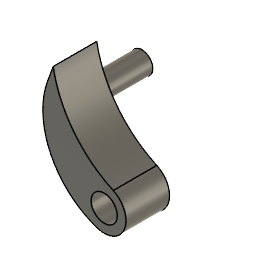
Pawl (Autodesk Fusion 360 design; units mm, degrees)
part number: 2026-05-26-15-53-21-879
Autodesk Fusion 360 part; units mm, degrees
sketch "ratchet scketch & pawl" plane through (0, 0, 0) normal (0, 1, 0) x (1, 0, 0)
  circle A0 centre (0, 0) radius 7.75 construction
  circle A1 centre (0, 0) radius 6.5 construction
  line L0 (0, 0) -> (1.3458, 7.6323) construction
  line L1 (0, 0) -> (-2.8494, 5.8422) construction
  arc A2 (1.3458, 7.6323) -> (-2.8494, 5.8422) centre (0.5379, 3.7147) ccw construction
  line L2 (0, 0) -> (6.5, 0) construction
  line L3 (0, 0) -> (4.4082, 25) construction
  circle A3 centre (2.9976, 17) radius 1.5
  circle A4 centre (2.9976, 17) radius 2.5
  line L4 (-2.8494, 5.8422) -> (-0.2045, 20.8422) construction
  line L5 (-2.8494, 5.8422) -> (-3.5335, 7.7215)
  arc A5 (4.0328, 14.7244) -> (-2.8494, 5.8422) centre (9.0259, 3.7482) ccw
  arc A6 (2.2215, 19.3765) -> (-3.5335, 7.7215) centre (5.0435, 10.7347) ccw
  circle A7 centre (-2.6702, 10.3422) radius 1.25
  dimension "d28" = 13
  dimension "d29" = 15.5
  dimension "d30" = 80
  dimension "d31" = 36
  dimension "d32" = 4
  dimension "d33" = 25
  dimension "d34" = 3
  dimension "d35" = 5
  dimension "d36" = 15
  dimension "d37" = 2
  dimension "d40" = 30
  dimension "d43" = 9.0909
  dimension "d44" = 17
  dimension "d45" = 2.5
  dimension "d46" = 4.5
  dimension "d47" = 7.7237
  constraint coincident A0.centre A1.centre
  constraint coincident A0 L0.end
  constraint coincident A1 L1.end
  constraint coincident A1 L2.end
  constraint horizontal L2
  constraint parallel L0 L3
  constraint coincident L3 A3.centre
  constraint concentric A3 A4
  constraint parallel L3 L4
  constraint tangent L4 A5
  constraint coincident A4 A5.start
  constraint coincident A4 A6.start
  constraint tangent A4 A5
  constraint tangent A4 A6
  measures "d28" diameter of A1
  measures "d29" diameter of A0
  measures "d30" angle of L0 L2
  measures "d31" angle of L0 L1
  measures "d32" radius of A2
  measures "d33" vertical distance of A0.centre L3.end
  measures "d34" diameter of A3
  measures "d35" diameter of A4
  measures "d36" vertical distance of L1.end L4.end
  measures "d37" distance of L1.end L5.end
  measures "d40" angle of L4 L5
  measures "d43" radius of A6
  measures "d44" vertical distance of A0.centre A3.centre
  measures "d45" diameter of A7
  measures "d46" vertical distance of L1.end A7.centre
  measures "d47" distance of A6.centre A7.centre
extrude "Extrude1" add sketch "ratchet scketch & pawl" along normal blind 5 contours A4 | A4 L5 A5 A6 | A7 makes body 1
move_body "Move1" bodies 1 to x (0, 0, 1) y (0, 1, 0) z (-1, 0, 0) at (-3.7668, 0, 14.8212)
extrude "Extrude2" add sketch "ratchet scketch & pawl" along normal blind 5 separate body contours A4 | A4 L5 A5 A6 | A7 makes body 2
extrude "Extrude3" add sketch "ratchet scketch & pawl" along normal blind 5 from surface at 5 contours A7 bodies 2
delete_body "RemoveBody1" bodies 1
equation "d29 = ( 7.75 * 2 ) * 1 mm"
named bodies: "pawl"
